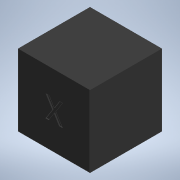
# Autodesk Inventor part: Cubo-0001-001
Saved by Autodesk Inventor 2020.1 (Build 241239000, 239)
## iProperties
Created: 2024-03-21
Part Number: Cubo-0001-001
Material: Rubber
Document SubType Name: Modeling
Designer: MiguelBarbosa
Density: 0.93 g/cm^3
Appearance: Rubber - Black
Author: MiguelBarbosa
## iProperties of the stored document _3DPrint.ipt
Created: 2024-03-21
Part Number: _3DPrint
Material: Generic
Document SubType Name: Modeling
Designer: MiguelBarbosa
Density: 1 g/cm^3
Appearance: Default
Author: MiguelBarbosa
Autodesk Inventor part; units mm, degrees
sketch "Sketch5" plane through (0, 0, 0) normal (0, 0, 1) x (1, 0, 0)
  line L0 (-20, -20) -> (20, -20)
  line L1 (20, -20) -> (20, 20)
  line L2 (20, 20) -> (-20, 20)
  line L3 (-20, 20) -> (-20, -20)
  line L4 (-20, -20) -> (20, 20) construction
  line L5 (20, -20) -> (-20, 20) construction
  point P0 (0, 0)
  dimension "d19" = 40
  constraints: 12 end point, 2 midpoint, 2 parallel, 2 perpendicular, 1 horizontal
  measures "d19" distance of L1.end L2.end
extrude "Extrusion5" add sketch "Sketch5" along normal mid plane 40
sketch "Sketch1" plane through (0, 0, 0) normal (0, 0, 1) x (1, 0, 0)
  line L0 (-25, -25) -> (25, -25)
  line L1 (25, -25) -> (25, 25)
  line L2 (25, 25) -> (-25, 25)
  line L3 (-25, 25) -> (-25, -25)
  line L4 (-25, -25) -> (25, 25) construction
  line L5 (25, -25) -> (-25, 25) construction
  point P0 (0, 0)
  dimension "d15" = 50
  dimension "d18" = 50
  constraints: 12 end point, 2 midpoint, 2 parallel, 1 horizontal, 1 perpendicular
  measures "d15" distance of L1.end L2.end
  measures "d18" distance of L2.end L0.start
extrude "Extrusion1" add sketch "Sketch1" along normal mid plane 50 separate body
sketch "Sketch2" plane through (0, 0, 25) normal (0, 0, 1) x (1, 0, 0)
  line L0 (-5.9866, 7.5) -> (5.9866, 7.5) construction
  line L1 (5.9866, 7.5) -> (5.9866, -7.5) construction
  line L2 (5.9866, -7.5) -> (-5.9866, -7.5) construction
  line L3 (-5.9866, -7.5) -> (-5.9866, 7.5) construction
  line L4 (-5.9866, 7.5) -> (5.9866, -7.5) construction
  line L5 (5.9015, -7.5) -> (3.6163, -7.5)
  line L6 (3.6163, -7.5) -> (-0.0304, -1.5194)
  line L7 (-0.0304, -1.5194) -> (-3.75, -7.5)
  line L8 (-3.75, -7.5) -> (-5.9015, -7.5)
  line L9 (-5.9015, -7.5) -> (-1.1244, 0.0122)
  line L10 (-1.1244, 0.0122) -> (-5.7557, 7.5)
  line L11 (-5.7557, 7.5) -> (-3.4704, 7.5)
  line L12 (-3.4704, 7.5) -> (0.1033, 1.6288)
  line L13 (0.1033, 1.6288) -> (3.75, 7.5)
  line L14 (3.75, 7.5) -> (5.9015, 7.5)
  line L15 (5.9015, 7.5) -> (1.2095, 0.1094)
  line L16 (1.2095, 0.1094) -> (5.9015, -7.5)
  point P0 (0, 0)
  point P1 (0, 0)
  point P2 (0, 0)
  point P3 (0, 0)
  dimension "d3" = 11.9733
  dimension "d4" = 15
  constraints: 3 coincident, 2 end point, 1 horizontal, 1 midpoint, 2 other
  measures "d3" distance of L0.start L0.end
  measures "d4" distance of L2.end L0.start
extrude "Extrusion2" cut sketch "Sketch2" against normal blind 0.6 bodies 2
sketch "Sketch7" plane through (-25, -25, 25) normal (-1, 0, 0) x (0, 0, 1)
  line L0 (-18.9344, 17.5) -> (-31.0656, 17.5) construction
  line L1 (-31.0656, 17.5) -> (-31.0656, 32.5) construction
  line L2 (-31.0656, 32.5) -> (-18.9344, 32.5) construction
  line L3 (-18.9344, 32.5) -> (-18.9344, 17.5) construction
  line L4 (-31.0656, 17.5) -> (-18.9344, 32.5) construction
  line L5 (-30.9562, 17.5) -> (-25.8874, 25.863)
  line L6 (-25.8874, 25.863) -> (-25.8874, 32.5)
  line L7 (-25.8874, 32.5) -> (-23.8938, 32.5)
  line L8 (-23.8938, 32.5) -> (-23.8938, 26.0697)
  line L9 (-23.8938, 26.0697) -> (-18.825, 17.5)
  line L10 (-18.825, 17.5) -> (-21.0373, 17.5)
  line L11 (-21.0373, 17.5) -> (-24.9028, 24.1005)
  line L12 (-24.9028, 24.1005) -> (-28.8412, 17.5)
  line L13 (-28.8412, 17.5) -> (-30.9562, 17.5)
  point P0 (-25, 25)
  point P1 (-25, 25)
  dimension "d27" = 12.1313
  dimension "d28" = 15
  constraints: 2 end point, 1 coincident, 1 horizontal, 1 midpoint, 2 other
  measures "d27" distance of L1.end L2.end
  measures "d28" distance of L0.end L1.end
extrude "Extrusion6" cut sketch "Sketch7" against normal blind 1 bodies 2
sketch "Sketch8" plane through (-25, -25, 25) normal (0, -1, 0) x (1, 0, 0)
  line L0 (19.2322, -17.5) -> (30.7678, -17.5) construction
  line L1 (30.7678, -17.5) -> (30.7678, -32.5) construction
  line L2 (30.7678, -32.5) -> (19.2322, -32.5) construction
  line L3 (19.2322, -32.5) -> (19.2322, -17.5) construction
  line L4 (25, -32.5) -> (25, -17.5) construction
  line L5 (30.3181, -32.5) -> (19.84, -32.5)
  line L6 (19.84, -32.5) -> (19.84, -30.6402)
  line L7 (19.84, -30.6402) -> (27.8626, -19.2747)
  line L8 (27.8626, -19.2747) -> (20.2046, -19.2747)
  line L9 (20.2046, -19.2747) -> (20.2046, -17.5)
  line L10 (20.2046, -17.5) -> (30.1114, -17.5)
  line L11 (30.1114, -17.5) -> (30.1114, -19.299)
  line L12 (30.1114, -19.299) -> (22.0036, -30.7253)
  line L13 (22.0036, -30.7253) -> (30.3181, -30.7253)
  line L14 (30.3181, -30.7253) -> (30.3181, -32.5)
  point P0 (25, -25)
  point P1 (25, -25)
  dimension "d31" = 15
  dimension "d32" = 11.5357
  constraints: 3 midpoint, 2 end point, 1 coincident, 1 horizontal, 2 other
  measures "d31" distance of L0.end L1.end
  measures "d32" distance of L0.start L0.end
extrude "Extrusion7" cut sketch "Sketch8" against normal blind 1 bodies 2
sketch "Sketch3" plane through (25, -25, 25) normal (1, 0, 0) x (0, 0, -1)
  line L0 (18.9344, 32.5) -> (31.0656, 32.5) construction
  line L1 (31.0656, 32.5) -> (31.0656, 17.5) construction
  line L2 (31.0656, 17.5) -> (18.9344, 17.5) construction
  line L3 (18.9344, 17.5) -> (18.9344, 32.5) construction
  line L4 (31.0656, 32.5) -> (18.9344, 17.5) construction
  point P0 (25, 25)
  point P1 (25, 25)
  dimension "d7" = 12.1313
  dimension "d8" = 15
  constraints: 2 end point, 1 coincident, 1 horizontal, 1 midpoint, 2 other
  measures "d7" distance of L0.start L0.end
  measures "d8" distance of L0.end L1.end
sketch "Sketch4" plane through (-25, 25, 25) normal (0, 1, 0) x (1, 0, 0)
  line L0 (19.2322, 32.5) -> (30.7678, 32.5) construction
  line L1 (30.7678, 32.5) -> (30.7678, 17.5) construction
  line L2 (30.7678, 17.5) -> (19.2322, 17.5) construction
  line L3 (19.2322, 17.5) -> (19.2322, 32.5) construction
  line L4 (30.7678, 32.5) -> (19.2322, 17.5) construction
  point P0 (25, 25)
  point P1 (25, 25)
  dimension "d11" = 11.5357
  dimension "d12" = 15
  constraints: 2 end point, 1 coincident, 1 horizontal, 1 midpoint, 2 other
  measures "d11" distance of L0.start L0.end
  measures "d12" distance of L0.end L1.end
equation "\"d20\" = d19"
equation "\"d18\" = d15"
equation "\"d1\" = d15"
body "Solid1"
body "Solid2"
